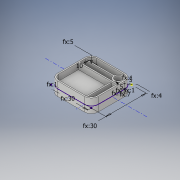
# Autodesk Inventor part: Base_part
Saved by Autodesk Inventor 2019.3 (Build 233278000, 278)
## iProperties
Created: 2019-01-28
Part Number: Base_part
Material: Generic
Document SubType Name: Modeling
Designer: Varga Daniel
Density: 1 g/cm^3
Appearance: Default
Outer_fillet: 5,000 mm
Inner_thickness: 1,000 mm
Hole_ring_thickness: 1,000 mm
Inner_route_thickness: 1,000 mm
Wall_thickness: 1,000 mm
Hole_diameter: 5,000 mm
Hole_diameter_toleracne: 0,000 mm
Overall_height: 10,000 mm
Hole_height: 8,400 mm
Width_tolerance: 0,000 mm
Length_tolerance: 0,000 mm
Author: Varga Daniel
Autodesk Inventor part; units mm, degrees
ref_plane "YZ Plane" through (0, 0, 0) normal (1, 0, 0) x (0, 1, 0)
ref_plane "XZ Plane" through (0, 0, 0) normal (0, 1, 0) x (-1, 0, 0)
ref_plane "XY Plane" through (0, 0, 0) normal (0, 0, 1) x (1, 0, 0)
sketch "Sketch1" plane through (0, 0, 0) normal (0, 1, 0) x (-1, 0, 0)
  line L0 (5, 0) -> (25, 0)
  line L1 (30, 5) -> (30, 25)
  line L2 (25, 30) -> (5, 30)
  line L3 (0, 25) -> (0, 5)
  line L4 (5, 29) -> (25, 29)
  line L5 (29, 25) -> (29, 5)
  line L6 (25, 1) -> (5, 1)
  line L7 (1, 5) -> (1, 25)
  circle A0 centre (5, 5) radius 2.5
  circle A1 centre (5, 5) radius 3.5
  arc A2 (25, 0) -> (30, 5) centre (25, 5) ccw
  arc A3 (30, 25) -> (25, 30) centre (25, 25) ccw
  arc A4 (5, 30) -> (0, 25) centre (5, 25) ccw
  arc A5 (0, 5) -> (5, 0) centre (5, 5) ccw
  arc A6 (1, 5) -> (5, 1) centre (5, 5) ccw
  arc A7 (5, 29) -> (1, 25) centre (5, 25) ccw
  arc A8 (29, 25) -> (25, 29) centre (25, 25) ccw
  arc A9 (25, 1) -> (29, 5) centre (25, 5) ccw
  line L8 (49.1041, 15) -> (-27.081, 15) construction
  line L9 (31.1478, 10) -> (-2.4877, 10) construction
  line L10 (-2.8604, 5) -> (35.495, 5) construction
  line L11 (5, -2.5736) -> (5, 36.7522) construction
  line L12 (15, -1.4978) -> (15, 34.8784) construction
  line L13 (1.5359, 5.5) -> (1, 5.5)
  line L14 (1.5359, 4.5) -> (1.0314, 4.5)
  line L15 (28.9686, 4.5) -> (8.4641, 4.5)
  line L16 (29, 5.5) -> (8.4641, 5.5)
  line L17 (4.5, 1.5359) -> (4.5, 1.0314)
  line L18 (5.5, 1.5359) -> (5.5, 1)
  line L19 (29, 10.5) -> (1, 10.5)
  line L20 (29, 9.5) -> (1, 9.5)
  line L21 (4.5, 28.9686) -> (4.5, 10.5)
  line L22 (4.5, 9.5) -> (4.5, 8.4641)
  line L23 (5.5, 29) -> (5.5, 10.5)
  line L24 (5.5, 9.5) -> (5.5, 8.4641)
  point P0 (0, 0)
  point P1 (30, 30)
  point P2 (0, 30)
  dimension "d46" = 7
  dimension "d0" = 30
  dimension "d1" = 30
  dimension "d2" = 1
  dimension "d3" = 5
  dimension "d5" = 5
  dimension "d7" = 5
  dimension "d8" = 4
  dimension "d29" = 5
  dimension "d40" = 10
  dimension "d58" = 1
  dimension "d59" = 1
  dimension "d72" = 1
  constraints: 50 end point, 20 point on circle, 20 point on line, 16 tangent, 9 centre point, 6 collinear, 6 equal radius, 6 horizontal, 6 parallel, 6 perpendicular, 4 vertical, 2 coincident, 18 other
  measures "d0" distance of point (0, 30) point (30, 30)
  measures "d1" distance between parallel lines of L0 L2
  measures "d2" distance between parallel lines of L4 L2
  measures "d3" diameter of A0
  measures "d5" distance from line of A0.centre L3
  measures "d7" radius of A2
  measures "d8" radius of A6
  measures "d29" distance from line of A0.centre L0
  measures "d40" distance between parallel lines of L9 L0
  measures "d58" distance between parallel lines of L13 L14
  measures "d59" distance between parallel lines of L17 L18
  measures "d72" distance between parallel lines of L19 L20
extrude "Extrusion5" add sketch "Sketch1" along normal blind 5 contours A5 L3 A4 L2 A3 L1 A2 L0 | L19 L5 L20 L7
extrude "Extrusion6" add sketch "Sketch1" against normal blind 5 contours A5 L3 A4 L2 A3 L1 A2 L0 | L19 L5 L20 L7
extrude "Extrusion7" add sketch "Sketch1" along normal blind 4.2 contours L4 L23 L19 L21 A7 | L5 A9 L15 A1 L16 | L24 A1 L22 L20 | L13 A1 L14 A6 L7 | A1 | L17 A1 L18 L6 A6
extrude "Extrusion8" add sketch "Sketch1" against normal blind 4.2 contours L4 L23 L19 L21 A7 | L5 A9 L15 A1 L16 | L24 A1 L22 L20 | L13 A1 L14 A6 L7 | A1 | L17 A1 L18 L6 A6
extrude "Extrusion9" add sketch "Sketch1" along normal blind 0.5 contours L4 A8 L5 L19 L23 | L21 L19 L7 A7 | L5 L16 A1 L24 L20 | L20 L22 A1 L13 L7 | A9 L6 L18 A1 L15 | L14 A1 L17 A6
extrude "Extrusion10" add sketch "Sketch1" against normal blind 0.5 contours L4 A8 L5 L19 L23 | L21 L19 L7 A7 | L5 L16 A1 L24 L20 | L20 L22 A1 L13 L7 | A9 L6 L18 A1 L15 | L14 A1 L17 A6
equation "\"d46\" = Hole_diameter + 2 * Wall_thickness"
equation "\"d2\" = Wall_thickness"
equation "\"d3\" = Hole_diameter + Hole_diameter_toleracne"
equation "\"d7\" = Outer_fillet"
equation "\"d8\" = Outer_fillet - Wall_thickness"
equation "\"Outer_fillet\" = 5"
equation "\"Hole_diameter\" = 5"
equation "\"Hole_diameter_toleracne\" = 0"
equation "\"Overall_height\" = 10"
equation "\"Inner_thickness\" = 1"
equation "\"Hole_ring_thickness\" = 1"
equation "\"Inner_route_thickness\" = 1"
equation "\"Wall_thickness\" = 1"
equation "\"Hole_height\" = 8.4"
equation "\"d52\" = Inner_route_thickness"
equation "\"d53\" = Inner_route_thickness"
equation "\"d54\" = Inner_route_thickness"
equation "\"Width_tolerance\" = 0"
equation "\"Length_tolerance\" = 0"
body "Solid4"
